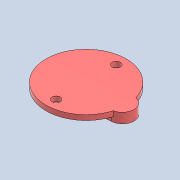
# Autodesk Inventor part: Thingy
Saved by Autodesk Inventor 2022 (Build 260153000, 153)
## iProperties
Created: 2023-02-26
Part Number: Thingy
Material: ABS Plastic
Document SubType Name: Modeling
Designer: byrne
Density: 1.06 g/cm^3
Appearance: Smooth - Red
Author: byrne
Autodesk Inventor part; units mm, degrees
ref_plane "YZ Plane" through (0, 0, 0) normal (1, 0, 0) x (0, 1, 0)
ref_plane "XZ Plane" through (0, 0, 0) normal (0, 1, 0) x (-1, 0, 0)
ref_plane "XY Plane" through (0, 0, 0) normal (0, 0, 1) x (1, 0, 0)
sketch "Sketch1" plane through (0, 0, 0) normal (0, 1, 0) x (-1, 0, 0)
  arc A0 (-0.2038, -3.7445) -> (-0.2038, 3.7445) centre (0, 0) ccw
  arc A1 (-23.1359, 2.4963) -> (-23.1359, -2.4963) centre (-23, 0) ccw
  line L0 (-0.2038, 3.7445) -> (-23.1359, 2.4963)
  line L1 (-23.1359, -2.4963) -> (-0.2038, -3.7445)
  line L2 (-23.3954, 7.2644) -> (-0.4633, 8.5126)
  arc A2 (-0.4633, -8.5126) -> (-0.4633, 8.5126) centre (0, 0) ccw
  line L3 (-0.4633, -8.5126) -> (-23.3954, -7.2644)
  arc A3 (-23.3954, 7.2644) -> (-23.3954, -7.2644) centre (-23, 0) ccw
  dimension "d0" = 7.5
  dimension "d25" = 5
  dimension "d26" = 23
  dimension "d27" = 4.7752
  constraints: 8 end point, 8 point on circle, 4 centre point, 4 tangent, 1 coincident, 1 horizontal alignment, 3 other
  measures "d0" diameter of A0
  measures "d25" diameter of A1
  measures "d26" distance of A1.centre A0.centre
  measures "d27" distance between parallel lines of L0 L2
extrude "Extrusion1" add sketch "Sketch1" along normal blind 3.175
sketch "Sketch2" plane through (0, 3.175, 0) normal (0, 1, 0) x (1, 0, 0)
  line L0 (-50.8, -50.8) -> (50.8, -50.8)
  line L1 (50.8, -50.8) -> (50.8, 50.8)
  line L2 (50.8, 50.8) -> (-50.8, 50.8)
  line L3 (-50.8, 50.8) -> (-50.8, -50.8)
  line L4 (47.625, 47.625) -> (47.625, -47.625)
  line L5 (47.625, -47.625) -> (-47.625, -47.625)
  line L6 (-47.625, -47.625) -> (-47.625, 47.625)
  line L7 (-47.625, 47.625) -> (47.625, 47.625)
  circle A0 centre (0, 0) radius 38.1 construction
  line L8 (-6.8036, -6.8036) -> (6.8036, -6.8036)
  line L9 (6.8036, -6.8036) -> (6.8036, 6.8036)
  line L10 (6.8036, 6.8036) -> (-6.8036, 6.8036)
  line L11 (-6.8036, 6.8036) -> (-6.8036, -6.8036)
  line L12 (-6.8036, -6.8036) -> (6.8036, 6.8036) construction
  line L13 (6.8036, -6.8036) -> (-6.8036, 6.8036) construction
  line L14 (18.368, -33.38) -> (0, 0)
  line L15 (0, 0) -> (-18.368, 33.38)
  line L16 (9.184, -16.69) -> (-32.398, -32.398)
  line L17 (-47.625, -47.625) -> (-32.398, -32.398)
  line L18 (47.625, 47.625) -> (32.398, 32.398)
  line L19 (-9.184, 16.69) -> (32.398, 32.398)
  line L20 (0.4633, -8.5126) -> (23.3954, -7.2644) projected
  arc A1 (23.3954, -7.2644) -> (23.3954, 7.2644) centre (23, 0) ccw projected
  line L21 (23.3954, 7.2644) -> (0.4633, 8.5126) projected
  arc A2 (0.4633, 8.5126) -> (0.4633, -8.5126) centre (0, 0) ccw projected
  line L22 (0.2038, 3.7445) -> (23.1359, 2.4963) projected
  arc A3 (23.1359, -2.4963) -> (23.1359, 2.4963) centre (23, 0) ccw projected
  line L23 (23.1359, -2.4963) -> (0.2038, -3.7445) projected
  arc A4 (0.2038, 3.7445) -> (0.2038, -3.7445) centre (0, 0) ccw projected
  point P0 (-47.625, 0)
  point P1 (0, -47.625)
  point P2 (-6.8036, 0)
  dimension "d4" = 101.6
  dimension "d5" = 101.6
  dimension "d6" = 3.175
  dimension "d7" = 76.2
  dimension "d12" = 13.6071
  dimension "d13" = 21.5342
  dimension "d14" = 21.5342
  dimension "d15" = 44.45
  constraints: 40 end point, 9 midpoint, 6 parallel, 3 perpendicular, 2 equal length, 2 horizontal, 2 horizontal alignment, 2 point on circle, 2 point on line, 1 centre point, 1 coincident, 1 vertical alignment, 3 other
  measures "d4" distance of L2.end L1.end
  measures "d5" distance of L1.end L0.end
  measures "d6" distance between parallel lines of L1 L4
  measures "d7" diameter of A0
  measures "d12" distance of L8.end L9.end
  measures "d13" distance of L5.end L16.end
  measures "d14" distance of L4.start L18.end
  measures "d15" distance of L16.start L16.end
sketch "Sketch3" plane through (0, 3.175, 0) normal (0, 1, 0) x (1, 0, 0)
  circle A0 centre (0, 0) radius 25.4
  circle A1 centre (0, -19.05) radius 2.6416
  circle A2 centre (0, 19.05) radius 2.6416
  line L0 (0, -19.05) -> (0, 19.05) construction
  line L1 (0.4633, -8.5126) -> (23.3954, -7.2644) projected
  arc A3 (23.3954, -7.2644) -> (23.3954, 7.2644) centre (23, 0) ccw projected
  line L2 (23.3954, 7.2644) -> (0.4633, 8.5126) projected
  arc A4 (0.4633, 8.5126) -> (0.4633, -8.5126) centre (0, 0) ccw projected
  line L3 (0.2038, 3.7445) -> (23.1359, 2.4963) projected
  arc A5 (23.1359, -2.4963) -> (23.1359, 2.4963) centre (23, 0) ccw projected
  line L4 (23.1359, -2.4963) -> (0.2038, -3.7445) projected
  arc A6 (0.2038, 3.7445) -> (0.2038, -3.7445) centre (0, 0) ccw projected
  point P0 (24.3746, -7.1442)
  point P1 (24.3746, 7.1442)
  dimension "d16" = 50.8
  dimension "d17" = 5.2832
  dimension "d18" = 38.1
  constraints: 3 centre point, 2 coincident, 2 end point, 1 equal radius, 1 midpoint, 1 vertical
  measures "d16" diameter of A0
  measures "d17" diameter of A1
  measures "d18" distance of L0.start L0.end
extrude "Extrusion2" add sketch "Sketch3" along normal blind 3.175
ref_plane "Work Plane1" through (-71.2155, 29.6, -71.2155) normal (0, 1, 0) x (-0.6077559, 0, 0.7941239)
equation "\"d12\" = d10"
equation "\"d14\" = d13"
equation "\"d10\" = 13.607143"
body "Solid1"
